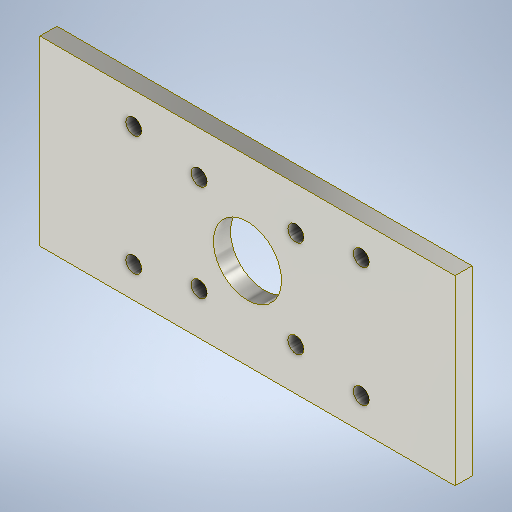
# Autodesk Inventor part: pequeño
Saved by Autodesk Inventor 2025.1 (Build 291241000, 241)
## iProperties
Created: 2024-12-02
Part Number: pequeño
Material: Stainless Steel
Document SubType Name: Modeling
Designer: Cristhian Vigo
Density: 8 g/cm^3
Appearance: Semi-Polished
Esla_Bas_Largo: 73.000 mm
Esla_Bas_Ancho: 32.000 mm
Esla_Bas_Espesor: 3.000 mm
Author: Cristhian Vigo
Autodesk Inventor part; units mm, degrees
ref_plane "YZ Plane" through (0, 0, 0) normal (1, 0, 0) x (0, 1, 0)
ref_plane "XZ Plane" through (0, 0, 0) normal (0, 1, 0) x (-1, 0, 0)
ref_plane "XY Plane" through (0, 0, 0) normal (0, 0, 1) x (1, 0, 0)
sketch "Sketch1" plane through (0, 0, 0) normal (0, 0, 1) x (1, 0, 0)
  line L0 (36.5, -16) -> (-36.5, -16)
  line L1 (-36.5, -16) -> (-36.5, 16)
  line L2 (-36.5, 16) -> (36.5, 16)
  line L3 (36.5, 16) -> (36.5, -16)
  line L4 (36.5, -16) -> (-36.5, 16) construction
  line L5 (-36.5, -16) -> (36.5, 16) construction
  point P0 (0, 0)
  dimension "Esla_Bas_Largo" = 73
  dimension "Esla_Bas_Ancho" = 32
  constraints: 12 end point, 2 midpoint, 2 parallel, 1 horizontal, 1 perpendicular
  measures "Esla_Bas_Largo" distance of L1.end L2.end
  measures "Esla_Bas_Ancho" distance of L2.end L0.start
extrude "Extrusion1" add sketch "Sketch1" along normal blind 3
sketch "Sketch2" plane through (0, 0, 3) normal (0, 0, 1) x (1, 0, 0)
  line L0 (24.0075, 15) -> (-24.0075, 15)
  line L1 (-24.0075, 15) -> (-24.0075, -15)
  line L2 (-24.0075, -15) -> (24.0075, -15)
  line L3 (24.0075, -15) -> (24.0075, 15)
  line L4 (24.0075, 15) -> (-24.0075, -15) construction
  line L5 (-24.0075, 15) -> (24.0075, -15) construction
  circle A0 centre (-20.0005, 10.5) radius 1.4
  circle A1 centre (-8.5005, 8.5) radius 1.4
  line L6 (0, 16.9064) -> (0, -19.8938) construction
  line L7 (-28.0201, 0) -> (28.1996, 0) construction
  circle A2 centre (20.0005, 10.5) radius 1.4
  circle A3 centre (8.5005, 8.5) radius 1.4
  circle A4 centre (-20.0005, -10.5) radius 1.4
  circle A5 centre (-8.5005, -8.5) radius 1.4
  circle A6 centre (8.5005, -8.5) radius 1.4
  circle A7 centre (20.0005, -10.5) radius 1.4
  circle A8 centre (0, 0) radius 6
  dimension "d4" = 48.015
  dimension "d5" = 30
  dimension "d6" = 4.007
  dimension "d7" = 4.5
  dimension "d8" = 2.8
  dimension "d9" = 2.8
  dimension "d10" = 6.5
  dimension "d11" = 15.507
  dimension "d14" = 12
  constraints: 16 end point, 9 centre point, 6 symmetric about line, 2 horizontal, 2 midpoint, 2 parallel, 1 coincident, 1 perpendicular, 1 vertical, 6 other
  measures "d4" distance of L2.end L1.end
  measures "d5" distance between parallel lines of L2 L0
  measures "d6" distance from line of A0.centre L1
  measures "d7" distance from line of A0.centre L0
  measures "d8" diameter of A0
  measures "d9" diameter of A1
  measures "d10" distance from line of L0 A1.centre
  measures "d11" distance from line of L1 A1.centre
  measures "d14" diameter of A8
extrude "Extrusion2" cut sketch "Sketch2" against normal through all contours A0 | A1 | A2 | A3 | A4 | A5 | A6 | A7 | A8
body "Solid1"
